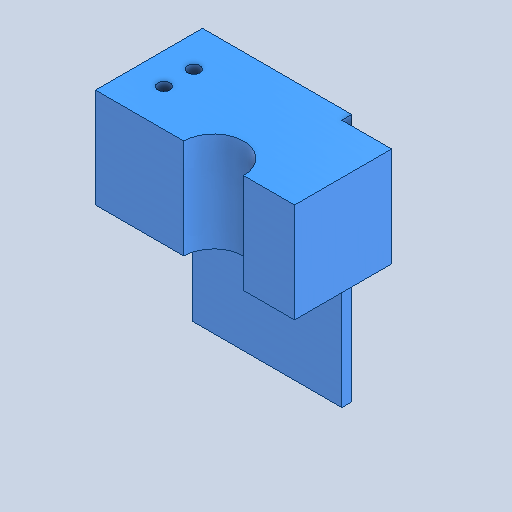
# Autodesk Inventor part: 主体
Saved by Autodesk Inventor 2022 (Build 260153000, 153)
## iProperties
Created: 2023-02-22
Part Number: 主体
Material: 常规
Document SubType Name: Modeling
Designer: 李承轩
Density: 1 g/cm^3
Appearance: 青色
Author: 李承轩
Autodesk Inventor part; units mm, degrees
ref_plane "YZ Plane" through (0, 0, 0) normal (1, 0, 0) x (0, 1, 0)
ref_plane "XZ Plane" through (0, 0, 0) normal (0, 1, 0) x (-1, 0, 0)
ref_plane "XY Plane" through (0, 0, 0) normal (0, 0, 1) x (1, 0, 0)
sketch "草图1" plane through (0, 0, 0) normal (0, 0, 1) x (1, 0, 0)
  line L0 (0, 0) -> (300, 0)
  line L1 (300, 0) -> (300, 500)
  line L2 (300, 500) -> (0, 500)
  line L3 (0, 500) -> (0, 0)
  line L4 (150, 500) -> (150, 0)
  circle A0 centre (62.5, 200) radius 20
  circle A1 centre (237.5, 200) radius 20
  dimension "d0" = 300
  dimension "d1" = 500
  dimension "d2" = 40
  dimension "d3" = 200
  dimension "d4" = 175
  constraints: 10 end point, 2 centre point, 2 midpoint, 2 parallel, 1 horizontal, 1 perpendicular, 1 symmetric about line, 1 other
  measures "d0" distance of L2.end L1.end
  measures "d1" distance of L1.end L0.end
  measures "d2" diameter of A0
  measures "d3" distance from line of L0 A0.centre
  measures "d4" distance of A0.centre A1.centre
extrude "拉伸1" add sketch "草图1" along normal blind 20
sketch "草图2" plane through (0, 0, 20) normal (0, 0, 1) x (1, 0, 0)
  line L0 (300, 500) -> (0, 500) construction
  line L1 (0, 500) -> (0, 0) construction
  line L2 (0, 0) -> (300, 0) construction
  line L3 (300, 0) -> (300, 500) construction
  circle A0 centre (62.5, 200) radius 20 construction
  circle A1 centre (237.5, 200) radius 20 construction
  line L4 (300, 500) -> (0, 500) projected
  line L5 (0, 500) -> (400, 500)
  line L6 (400, 500) -> (400, 300)
  line L7 (400, 300) -> (0, 300)
  line L8 (0, 300) -> (0, 500)
  dimension "d7" = 400
  dimension "d8" = 200
  constraints: 8 end point, 2 parallel, 1 horizontal, 1 perpendicular
  measures "d7" distance of L6.end L7.end
  measures "d8" distance of L5.end L6.end
extrude "拉伸2" add sketch "草图2" along normal blind 195
sketch "草图3" plane through (0, 500, 0) normal (0, 1, 0) x (1, 0, 0)
  line L0 (237.5, 53) -> (237.5, -318) projected
  line L1 (300, 0) -> (0, 0) construction
  line L2 (0, 0) -> (0, -215) construction
  line L3 (400, -215) -> (0, -215) construction
  line L4 (400, -20) -> (400, -215) construction
  line L5 (400, -20) -> (300, -20) construction
  line L6 (300, 0) -> (300, -20) construction
  line L7 (0, -215) -> (400, -215) projected
  circle A0 centre (237.5, -215) radius 60
  dimension "d11" = 120
  constraints: 2 point on line, 1 centre point
  measures "d11" diameter of A0
extrude "拉伸3" cut sketch "草图3" against normal through all
sketch "草图4" plane through (0, 500, 0) normal (0, 1, 0) x (1, 0, 0)
  line L0 (62.5, 43) -> (62.5, -258) projected
  arc A0 (297.5, -215) -> (177.5, -215) centre (237.5, -215) ccw construction
  line L1 (0, -215) -> (177.5, -215) construction
  line L2 (0, -20) -> (0, -215) construction
  line L3 (300, -20) -> (0, -20) construction
  line L4 (300, -20) -> (400, -20) construction
  line L5 (400, -20) -> (400, -215) construction
  line L6 (297.5, -215) -> (400, -215) construction
  point P0 (0, 0)
  point P1 (62.5, -80)
  point P2 (62.5, -140)
  dimension "d14" = 60
  dimension "d15" = 60
  constraints: 2 point on line
  measures "d14" distance from line of L3 point (62.5, -80)
  measures "d15" distance of point (62.5, -140) point (62.5, -80)
hole "孔1" at (62.5, 500, 80) at (62.5, 500, 140) direction (0, -1, 0) diameter 25 end through all
sketch "草图5" plane through (0, 0, 0) normal (0, -1, 0) x (1, 0, 0)
  line L0 (0, 0) -> (300, 0) construction
  line L1 (300, 0) -> (300, 20) construction
  line L2 (0, 20) -> (300, 20) construction
  line L3 (0, 0) -> (0, 20) construction
  line L4 (300, 0) -> (0, 0) projected
  line L5 (150, 0) -> (150, 100)
  line L6 (150, 0) -> (250, 0) construction
  line L7 (300, 20) -> (0, 20) construction
  line L8 (40, 20) -> (60, 20)
  line L9 (60, 20) -> (60, -30)
  line L10 (60, -30) -> (40, -30)
  line L11 (40, -30) -> (40, 20)
  line L12 (260, 20) -> (240, 20)
  line L13 (240, 20) -> (240, -30)
  line L14 (240, -30) -> (260, -30)
  line L15 (260, -30) -> (260, 20)
  dimension "d23" = 100
  dimension "d24" = 90
  dimension "d25" = 300
  dimension "d26" = 20
  dimension "d27" = 50
  dimension "d28" = 180
  constraints: 20 end point, 4 symmetric about line, 3 perpendicular, 2 horizontal, 2 parallel, 1 midpoint, 1 point on line
  measures "d23" distance of L5.start L5.end
  measures "d24" angle of L6 L5
  measures "d25" diameter of L4.end L5
  measures "d26" distance of L9.end L10.end
  measures "d27" distance of L8.end L9.end
  measures "d28" distance between parallel lines of L13 L9
extrude "拉伸4" add sketch "草图5" against normal blind 10
full round fillet "全圆角1" first side at (60, 3.3333, -20) centre faces at (46.6667, 3.3333, -30) second side at (40, 3.3333, -10)
full round fillet "全圆角2" first side at (260, 3.3333, -20) centre faces at (246.6667, 3.3333, -30) second side at (240, 3.3333, -10)
sketch "草图6" plane through (0, 10, 0) normal (0, 1, 0) x (1, 0, 0)
  arc A0 (260, 20) -> (240, 20) centre (250, 20) ccw projected
  point P0 (0, 0)
  point P1 (50.1604, 17.9561)
  constraints: 1 coincident
hole "孔2" at (50.1604, 10, -17.9561) at (250, 10, -20) direction (0, -1, 0) diameter 10 end through all
